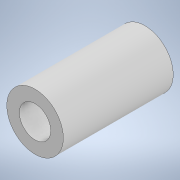
# Autodesk Inventor part: tuleja_M5_M9_17.5
Saved by Autodesk Inventor 2020.3 (Build 243373000, 373)
## iProperties
Created: 2021-11-02
Part Number: tuleja_M5_M9_17.5
Material: Ogólny
Document SubType Name: Modeling
Designer: patry
Density: 1 g/cm^3
Appearance: Domyślna
Author: patry
Autodesk Inventor part; units mm, degrees
ref_plane "YZ Plane" through (0, 0, 0) normal (1, 0, 0) x (0, 1, 0)
ref_plane "XZ Plane" through (0, 0, 0) normal (0, 1, 0) x (-1, 0, 0)
ref_plane "XY Plane" through (0, 0, 0) normal (0, 0, 1) x (1, 0, 0)
sketch "Szkic1" plane through (0, 0, 0) normal (0, 0, 1) x (1, 0, 0)
  circle A0 centre (0, 0) radius 2.5
  circle A1 centre (0, 0) radius 4.5
  dimension "d0" = 5
  dimension "d1" = 9
  constraints: 2 centre point, 2 coincident
  measures "d0" diameter of A0
  measures "d1" diameter of A1
extrude "Wyciągnięcie proste1" add sketch "Szkic1" along normal blind 17.5
